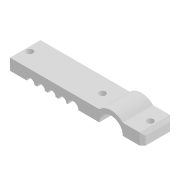
# Autodesk Inventor part: C_Unit_Cable_Holder_A
Saved by Autodesk Inventor 2020 (Build 240168000, 168)
## iProperties
Created: 2021-02-20
Part Number: C_Unit_Cable_Holder_A
Material: 一般
Document SubType Name: Modeling
Designer: ken113
Density: 1 g/cm^3
Appearance: 既定
Author: ken113
Autodesk Inventor part; units mm, degrees
ref_plane "YZ Plane" through (0, 0, 0) normal (1, 0, 0) x (0, 1, 0)
ref_plane "XZ Plane" through (0, 0, 0) normal (0, 1, 0) x (-1, 0, 0)
ref_plane "XY Plane" through (0, 0, 0) normal (0, 0, 1) x (1, 0, 0)
sketch "スケッチ1" plane through (0, 0, 0) normal (0, 0, 1) x (1, 0, 0)
  circle A0 centre (0, 9) radius 7.75
  line L0 (10.75, 0) -> (-58.5, 0)
  line L1 (-58.5, 0) -> (-58.5, 1.25)
  line L2 (-58.5, 1.25) -> (10.75, 1.25)
  line L3 (10.75, 1.25) -> (10.75, 0)
  circle A1 centre (0, 9) radius 10.75
  line L4 (10.75, 1.25) -> (10.75, 15.8822)
  circle A2 centre (-32, 9) radius 2.5
  circle A3 centre (-39, 9) radius 2.5
  circle A4 centre (-25, 9) radius 3.5
  circle A5 centre (-46, 9) radius 2.5
  circle A6 centre (-53, 9) radius 2.5
  circle A7 centre (-53, 9) radius 5.5
  line L5 (-58.5, 1.25) -> (-58.5, 18.7354)
  line L6 (-61.6708, 14.5) -> (12.7388, 14.5)
  point P0 (0, 0)
  point P1 (-9.2365, 14.5)
  point P2 (-58.5, 14.5)
  point P3 (10.75, 14.5)
  point P4 (9.2365, 14.5)
  dimension "d0" = 15.5
  dimension "d1" = 3
  dimension "d2" = 5
  dimension "d3" = 5
  dimension "d4" = 7
  dimension "d5" = 5
  dimension "d7" = 7
  dimension "d8" = 7
  dimension "d9" = 25
  dimension "d10" = 7
  dimension "d11" = 5
  dimension "d12" = 7
  dimension "d13" = 3
  dimension "d16" = 9
  constraints: 14 end point, 8 centre point, 6 horizontal alignment, 6 tangent, 2 parallel, 2 perpendicular, 1 horizontal, 1 vertical alignment
  measures "d0" diameter of A0
  measures "d1" radial gap between concentric circles of A0 A1
  measures "d2" diameter of A2
  measures "d3" diameter of A3
  measures "d4" diameter of A4
  measures "d5" diameter of A5
  measures "d7" distance of A2.centre A3.centre
  measures "d8" distance of A5.centre A3.centre
  measures "d9" distance of A0.centre A4.centre
  measures "d10" distance of A4.centre A2.centre
  measures "d11" diameter of A6
  measures "d12" distance of A6.centre A5.centre
  measures "d13" radial gap between concentric circles of A6 A7
  measures "d16" distance from line of A4.centre L0
extrude "押し出し1" add sketch "スケッチ1" along normal blind 20 contours A0 L6 A1 L2 | A0 L6 A1 | L2 A1 L6 A0 | L2 A1 L0 | L6 L4 A1 | A1 L0 L1 L2 | L2 L5 A7 A5 L6 A1 | A1 L4 L2 | L2 L3 L0 A1 | A7 A5 | A7 L5 L6 picked at (-49.0972, 10.8197)
sketch "スケッチ3" plane through (0, 0, 20) normal (0, 0, 1) x (1, 0, 0)
  line L0 (-9.2365, 14.5) -> (-58.5, 14.5) projected
  line L1 (-58.5, 14.5) -> (-58.5, 0) projected
  line L2 (-58.5, 0) -> (10.75, 0) projected
  line L3 (10.75, 0) -> (10.75, 14.5) projected
  line L4 (10.75, 14.5) -> (9.2365, 14.5) projected
  arc A0 (9.2365, 14.5) -> (-9.2365, 14.5) centre (0, 9) ccw projected
  circle A1 centre (0, 9) radius 7.75 projected
  circle A2 centre (-53, 9) radius 2.5 projected
  circle A3 centre (-25, 9) radius 3.5 projected
  circle A4 centre (-39, 9) radius 2.5 projected
  circle A5 centre (-32, 9) radius 2.5 projected
  circle A6 centre (-46, 9) radius 2.5 projected
  line L5 (-58.5, 14.5) -> (-58.5, 0) projected
  line L6 (-58.5, 0) -> (-68.5, 0)
  line L7 (-68.5, 0) -> (-68.5, 14.5)
  line L8 (-68.5, 14.5) -> (-58.5, 14.5)
  line L9 (-58.5, 14.5) -> (-58.5, 0)
  line L10 (10.75, 0) -> (20.75, 0)
  line L11 (20.75, 0) -> (20.75, 14.5)
  line L12 (20.75, 14.5) -> (10.75, 14.5)
  line L13 (10.75, 14.5) -> (10.75, 0)
  point P0 (0, 0)
  dimension "d17" = 10
  dimension "d18" = 10
  constraints: 16 end point, 4 parallel, 2 horizontal, 2 perpendicular, 1 coincident, 1 horizontal alignment
  measures "d17" distance of L7.end L8.end
  measures "d18" distance of L11.end L12.end
extrude "押し出し2" add sketch "スケッチ3" against normal up to surface (20 mm away) contours L1 L6 L7 L8 | L12 L11 L10 L3
sketch "スケッチ4" plane through (0, 0, 20) normal (0, 0, 1) x (1, 0, 0)
  line L0 (-9.2365, 14.5) -> (-68.5, 14.5) projected
  line L1 (-68.5, 14.5) -> (-68.5, 0) projected
  line L2 (-68.5, 0) -> (20.75, 0) projected
  line L3 (20.75, 0) -> (20.75, 14.5) projected
  line L4 (20.75, 14.5) -> (9.2365, 14.5) projected
  arc A0 (9.2365, 14.5) -> (-9.2365, 14.5) centre (0, 9) ccw projected
  circle A1 centre (0, 9) radius 7.75 projected
  circle A2 centre (-53, 9) radius 2.5 projected
  circle A3 centre (-25, 9) radius 3.5 projected
  circle A4 centre (-39, 9) radius 2.5 projected
  circle A5 centre (-32, 9) radius 2.5 projected
  circle A6 centre (-46, 9) radius 2.5 projected
  line L5 (-68.5, 0) -> (-68.5, 14.5) projected
  line L6 (20.75, 0) -> (20.75, 14.5) projected
  line L7 (-68.5, 0) -> (20.75, 0)
  line L8 (20.75, 0) -> (20.75, 9)
  line L9 (20.75, 9) -> (-68.5, 9)
  line L10 (-68.5, 9) -> (-68.5, 0)
  point P0 (0, 0)
  point P1 (-55.5, 9)
  point P2 (-68.5, 9)
  point P3 (7.75, 9)
  point P4 (-7.75, 9)
  point P5 (-28.5, 9)
  point P6 (-21.5, 9)
  point P7 (-29.5, 9)
  point P8 (-34.5, 9)
  point P9 (-36.5, 9)
  point P10 (-41.5, 9)
  point P11 (-43.5, 9)
  point P12 (-48.5, 9)
  point P13 (-50.5, 9)
  constraints: 8 end point, 2 parallel, 1 horizontal, 1 horizontal alignment, 1 perpendicular, 1 point on line
extrude "押し出し3" cut sketch "スケッチ4" against normal through all contours L9 A2 A6 A4 A5 A3 A1 L3 L2 L1 | L9 A3 | A3 L9
sketch "スケッチ6" plane through (0, 0, 20) normal (0, 0, 1) x (1, 0, 0)
  line L0 (-43.5, 9) -> (-41.5, 9) projected
  arc A0 (-36.5, 9) -> (-41.5, 9) centre (-39, 9) ccw projected
  line L1 (-36.5, 9) -> (-34.5, 9) projected
  arc A1 (-29.5, 9) -> (-34.5, 9) centre (-32, 9) ccw projected
  line L2 (-29.5, 9) -> (-28.5, 9) projected
  arc A2 (-21.5, 9) -> (-28.5, 9) centre (-25, 9) ccw projected
  line L3 (-21.5, 9) -> (-7.75, 9) projected
  arc A3 (7.75, 9) -> (-7.75, 9) centre (0, 9) ccw projected
  line L4 (7.75, 9) -> (20.75, 9) projected
  line L5 (20.75, 9) -> (20.75, 14.5) projected
  line L6 (20.75, 14.5) -> (9.2365, 14.5) projected
  arc A4 (9.2365, 14.5) -> (-9.2365, 14.5) centre (0, 9) ccw projected
  line L7 (-9.2365, 14.5) -> (-68.5, 14.5) projected
  line L8 (-68.5, 14.5) -> (-68.5, 9) projected
  line L9 (-68.5, 9) -> (-55.5, 9) projected
  arc A5 (-50.5, 9) -> (-55.5, 9) centre (-53, 9) ccw projected
  line L10 (-50.5, 9) -> (-48.5, 9) projected
  arc A6 (-43.5, 9) -> (-48.5, 9) centre (-46, 9) ccw projected
  line L11 (-68.5, 14.5) -> (20.75, 14.5)
  line L12 (20.75, 14.5) -> (20.75, 16.5)
  line L13 (20.75, 16.5) -> (-68.5, 16.5)
  line L14 (-68.5, 16.5) -> (-68.5, 14.5)
  point P0 (0, 0)
  point P1 (7.7015, 16.5)
  point P2 (-7.7015, 16.5)
  dimension "d33" = 2
  constraints: 8 end point, 2 parallel, 1 horizontal, 1 perpendicular, 1 vertical alignment
  measures "d33" distance of L13.end L7.end
extrude "押し出し4" add sketch "スケッチ6" against normal up to surface (20 mm away) contours L14 L13 A4 L7 | L13 L12 L6 A4
sketch "スケッチ7" plane through (7.7015, 16.5, 20) normal (0, 1, 0) x (1, 0, 0)
  line L0 (0, 20) -> (13.0485, 20) projected
  line L1 (0, 0) -> (0, 20) projected
  line L2 (13.0485, 0) -> (0, 0) projected
  line L3 (13.0485, 0) -> (13.0485, 20) projected
  line L4 (-76.2015, 20) -> (-15.4029, 20) projected
  line L5 (-76.2015, 0) -> (-76.2015, 20) projected
  line L6 (-15.4029, 0) -> (-76.2015, 0) projected
  line L7 (-15.4029, 20) -> (-15.4029, 0) projected
  point P0 (-7.7015, 20)
  point P1 (8.0485, 10)
  point P2 (-23.4515, 10)
  point P3 (-71.2015, 10)
  dimension "d36" = 5
  dimension "d37" = 10
  dimension "d38" = 10
  dimension "d39" = 15.75
  dimension "d40" = 5
  constraints: 1 horizontal alignment
  measures "d36" distance from line of L3 point (8.049, 10)
  measures "d37" distance from line of L2 point (8.049, 10)
  measures "d38" distance from line of L6 point (-71.201, 10)
  measures "d39" horizontal distance of point (-23.451, 10) point (-7.701, 20)
  measures "d40" distance from line of L5 point (-71.201, 10)
hole "穴2" at (15.75, 16.5, 10) at (-15.75, 16.5, 10) at (-63.5, 16.5, 10) direction (0, -1, 0) diameter 4.3 end through all
chamfer "面取り1" distance 2 angle 45 2 edges at (20.75, 16.5, 10) (-68.5, 16.5, 10)
chamfer "面取り2" distance 2 angle 45 4 edges at (20.75, 11.75, 0) (20.75, 11.75, 20) (-68.5, 11.75, 0) (-68.5, 11.75, 20)
